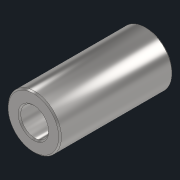
# Autodesk Inventor part: CF-417E
Saved by Autodesk Inventor 2022 (Build 260153000, 153)
## iProperties
Created: 2021-09-17
Part Number: CF-417E
Material: 鋼、炭素鋼
Document SubType Name: Modeling
Designer: Yuta Kage
Density: 7.85 g/cm^3
Appearance: 半つや出し
Author: Yuta Kage
Autodesk Inventor part; units mm, degrees
ref_plane "YZ Plane" through (0, 0, 0) normal (1, 0, 0) x (0, 1, 0)
ref_plane "XZ Plane" through (0, 0, 0) normal (0, 1, 0) x (-1, 0, 0)
ref_plane "XY Plane" through (0, 0, 0) normal (0, 0, 1) x (1, 0, 0)
sketch "スケッチ1" plane through (0, 0, 0) normal (0, 0, 1) x (1, 0, 0)
  circle A0 centre (0, 0) radius 2.1
  circle A1 centre (0, 0) radius 4
  dimension "d0" = 4.2
  dimension "d1" = 8
  constraints: 2 centre point, 2 coincident
  measures "d0" diameter of A0
  measures "d1" diameter of A1
extrude "押し出し1" add sketch "スケッチ1" along normal mid plane 17
chamfer "面取り1" distance 0.2 angle 45 4 edges at (-2.1, 0, 8.5) (-4, 0, 8.5) (-4, 0, -8.5) (-2.1, 0, -8.5)
